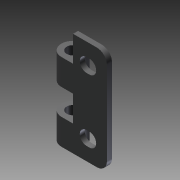
# Autodesk Inventor part: SHPSNA5_2
Saved by Autodesk Inventor 2015 SP1 (Build 190203100, 203)
## iProperties
Category: PARTsolutions
Company: MISUMI
Created: 2015-01-26
Part Number: SHPSNA5_2
Catalog Web Link: www.cadenas.de
Description: SHPSNA_2-Hinges with Slotted Holes
Vendor: MISUMI
Document SubType Name: Modeling
Designer: PARTuser1
Manufacturer: MISUMI
Mass: 2.00758 g
Surface Area: 23.5157 cm^2
Volume: 2.00758 cm^3
Density: 1 g/cm^3
Material: Generic
Appearance: PSOLRGB-192-192-192
PSOL_IDENT_0: {\\10.0.0.236\data_v8\23d-libs\misumi\metric\44_handles_hinges\shpsna_2.prj},162 {VTYP=3D},{NB=SHPSN
PSOL_IDENT_1: A5_2},{LINA=SHPSNA5_2},{NN=SHPSNA_2},{DATE=14.11.2014 09:15:25},{GEOMDATE=31.03.2009 09:23:00},{VERS
PSOL_IDENT_2: ION=},{LINEID=10},{LINESUBID=-1},{WBVAR=}  {NB=SHPSNA5_2},{LINA=SHPSNA5_2},{KT=DUMMY},{PN=SHPSNA5},{
PSOL_IDENT_3: TYPE=SHPSNA},{MAT=304 Stainless Steel},{NO=5},{AL1=9},{AL2=88},{MASS=43},{L=41},{W=36},{K=8},{P=25},
PSOL_IDENT_4: {J=7.5},{S=21},{N=5.5},{Z=5.5x6.5},{Z1=5.5},{Z2=6.5},{T=2},{E=4.6},{R=4.6},{CR=4},{D=5}
SUPPLIER: MISUMI
ARTICLENO: SHPSNA5_2
BOMINFO: SHPSNA5_2
CREATOR: CADENAS GmbH
Title: SHPSNA5_2
Author: Cadenas PARTsolutions
Comments: Hinges with Slotted Holes
Autodesk Inventor part; units mm, degrees
sketch "Sketch_1" plane through (0, 0, 0) normal (0, 0, 1) x (1, 0, 0)
  arc A0 (3.7947, -2.6) -> (0, -4.6) centre (0, 0) ccw
  line L0 (0, -4.6) -> (18, -4.6)
  line L1 (18, -4.6) -> (18, -2.6)
  line L2 (18, -2.6) -> (3.7947, -2.6)
  circle A1 centre (0, 0) radius 2.5
  constraints: 6 end point, 2 centre point, 2 point on circle
extrude "Extrusion1" add sketch "Sketch_1" along normal blind 41
sketch "Sketch_2" plane through (0, -4.6, 0) normal (0, 1, 0) x (1, 0, 0)
  line L0 (9.2, -41) -> (9.2, -43)
  line L1 (9.2, -43) -> (20, -43)
  line L2 (20, -43) -> (20, 2)
  line L3 (20, 2) -> (9.2, 2)
  line L4 (9.2, 2) -> (9.2, 0)
  line L5 (9.2, 0) -> (14, 0)
  arc A0 (18, -4) -> (14, 0) centre (14, -4) ccw
  line L6 (18, -4) -> (18, -37)
  arc A1 (14, -41) -> (18, -37) centre (14, -37) ccw
  line L7 (14, -41) -> (9.2, -41)
  constraints: 16 end point, 4 point on circle, 2 centre point
extrude "Extrusion2" cut sketch "Sketch_2" along normal blind 2
sketch "Sketch_7" plane through (0, 0, 20.5) normal (0, 0, 1) x (1, 0, 0)
  arc A0 (4.6, 0) -> (0, -4.6) centre (0, 0) ccw
  line L0 (0, -4.6) -> (4.6, -4.6)
  line L1 (4.6, -4.6) -> (4.6, 0)
  constraints: 4 end point, 2 point on circle, 1 centre point
extrude "Extrusion3" cut sketch "Sketch_7" against normal blind 10.25
sketch "Sketch_5" plane through (0, 0, 41) normal (0, 0, 1) x (1, 0, 0)
  arc A0 (4.6, 0) -> (0, -4.6) centre (0, 0) ccw
  line L0 (0, -4.6) -> (4.6, -4.6)
  line L1 (4.6, -4.6) -> (4.6, 0)
  constraints: 4 end point, 2 point on circle, 1 centre point
extrude "Extrusion4" cut sketch "Sketch_5" against normal blind 10.25
sketch "Sketch_3" plane through (0, -4.6, 0) normal (0, 1, 0) x (1, 0, 0)
  arc A0 (10, -5.25) -> (10, -10.75) centre (10, -8) ccw
  line L0 (10, -10.75) -> (11, -10.75)
  arc A1 (11, -10.75) -> (11, -5.25) centre (11, -8) ccw
  line L1 (11, -5.25) -> (10, -5.25)
  constraints: 4 end point, 4 point on circle, 2 centre point
extrude "Extrusion5" cut sketch "Sketch_3" along normal blind 2
sketch "Sketch_4" plane through (0, -4.6, 0) normal (0, 1, 0) x (1, 0, 0)
  arc A0 (10, -30.25) -> (10, -35.75) centre (10, -33) ccw
  line L0 (10, -35.75) -> (11, -35.75)
  arc A1 (11, -35.75) -> (11, -30.25) centre (11, -33) ccw
  line L1 (11, -30.25) -> (10, -30.25)
  constraints: 4 end point, 4 point on circle, 2 centre point
extrude "Extrusion6" cut sketch "Sketch_4" along normal blind 2
ref_plane "2_to_1_XY" through (0, 0, 20.5) normal (0, 0, 1) x (1, 0, 0)
ref_plane "2_to_1_YZ" through (0, 0, 20.5) normal (1, 0, 0) x (0, 1, 0)
ref_plane "2_to_1_ZX" through (0, 0, 20.5) normal (0, 1, 0) x (0, 0, 1)
body "Solid1"
